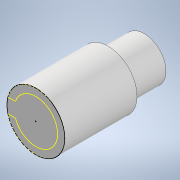
# Autodesk Inventor part: handle_base3
Saved by Autodesk Inventor 2021 (Build 250183000, 183)
## iProperties
Created: 2021-07-05
Part Number: handle_base3
Material: Generic
Document SubType Name: Modeling
Designer: teh18
Density: 1 g/cm^3
Appearance: Default
Author: teh18
Autodesk Inventor part; units mm, degrees
ref_plane "YZ Plane" through (0, 0, 0) normal (1, 0, 0) x (0, 1, 0)
ref_plane "XZ Plane" through (0, 0, 0) normal (0, 1, 0) x (-1, 0, 0)
ref_plane "XY Plane" through (0, 0, 0) normal (0, 0, 1) x (1, 0, 0)
sketch "Sketch1" plane through (0, 0, 0) normal (0, 0, 1) x (1, 0, 0)
  circle A0 centre (0, 0) radius 6.1 projected
  circle A1 centre (0, 0) radius 8 projected
  circle A2 centre (0, 0) radius 6.1 projected
  circle A3 centre (0, 0) radius 6
  circle A4 centre (-0.2369, 0.08) radius 5 projected
  circle A5 centre (-0.2369, 0.08) radius 5 projected
  point P0 (0, 0)
  dimension "d0" = 0.1
  constraints: 1 centre point
  measures "d0" radial gap between concentric circles of A0 A3
extrude "Extrusion1" add sketch "Sketch1" against normal blind 10 contours A3
sketch "Sketch2" plane through (0, 0, 0) normal (0, 0, 1) x (1, 0, 0)
  circle A0 centre (0, 0) radius 6.1 projected
  circle A1 centre (0, 0) radius 8 projected
  circle A2 centre (0, 0) radius 6 projected
  point P0 (0, 0)
extrude "Extrusion2" add sketch "Sketch2" along normal blind 20 contours A0 | A1
sketch "Sketch3" plane through (0, 0, 20) normal (0, 0, 1) x (1, 0, 0)
  line L0 (-1.3404, -2) -> (-8, -2)
  line L1 (-8, -2) -> (-8, 2)
  line L2 (-8, 2) -> (-1.3404, 2)
  line L3 (-1.3404, 2) -> (-1.3404, -2)
  line L4 (-1.3404, -2) -> (-8, 2) construction
  line L5 (-8, -2) -> (-1.3404, 2) construction
  point P0 (0, 0)
  point P1 (-4.6702, 0)
  dimension "d5" = 4
  constraints: 12 end point, 2 midpoint, 2 parallel, 1 horizontal, 1 perpendicular
  measures "d5" distance of L0.end L1.end
extrude "Extrusion3" cut sketch "Sketch3" against normal blind 7
sketch "Sketch4" plane through (0, 0, 20) normal (0, 0, 1) x (1, 0, 0)
  line L0 (-5.6569, -2) -> (-7.746, -2) projected
  arc A0 (-7.746, -2) -> (-7.746, 2) centre (0, 0) ccw projected
  line L1 (-7.746, 2) -> (-5.6569, 2) projected
  arc A1 (-5.6569, -2) -> (-5.6569, 2) centre (0, 0) ccw projected
  circle A2 centre (0, 0) radius 8
  point P0 (0, 0)
  point P1 (-7.746, 2)
  constraints: 1 centre point, 1 coincident, 1 concentric
extrude "Extrusion4" add sketch "Sketch4" against normal blind 3
sketch "Sketch6" plane through (0, 0, 20) normal (0, 0, 1) x (1, 0, 0)
  circle A0 centre (0, 0) radius 8 projected
  arc A1 (-4.1289, 4.2146) -> (-5.6926, 1.5507) centre (0, 0) ccw projected
  line L0 (-5.6926, 1.5507) -> (-7.0866, 0.985) projected
  line L1 (-7.0866, 0.985) -> (-5.8997, 0.0606) projected
  arc A2 (-5.8997, 0.0606) -> (-5.1217, -2.9288) centre (0, 0) ccw projected
  line L2 (-5.1217, -2.9288) -> (-5.7075, -4.3145) projected
  line L3 (-5.7075, -4.3145) -> (-4.2146, -4.1289) projected
  arc A3 (-4.2146, -4.1289) -> (-1.5507, -5.6926) centre (0, 0) ccw projected
  line L4 (-1.5507, -5.6926) -> (-0.985, -7.0866) projected
  line L5 (-0.985, -7.0866) -> (-0.0606, -5.8997) projected
  arc A4 (-0.0606, -5.8997) -> (2.9288, -5.1217) centre (0, 0) ccw projected
  line L6 (2.9288, -5.1217) -> (4.3145, -5.7075) projected
  line L7 (4.3145, -5.7075) -> (4.1289, -4.2146) projected
  arc A5 (4.1289, -4.2146) -> (5.6926, -1.5507) centre (0, 0) ccw projected
  line L8 (5.6926, -1.5507) -> (7.0866, -0.985) projected
  line L9 (7.0866, -0.985) -> (5.8997, -0.0606) projected
  arc A6 (5.8997, -0.0606) -> (5.1217, 2.9288) centre (0, 0) ccw projected
  line L10 (5.1217, 2.9288) -> (5.7075, 4.3145) projected
  line L11 (5.7075, 4.3145) -> (4.2146, 4.1289) projected
  arc A7 (4.2146, 4.1289) -> (1.5507, 5.6926) centre (0, 0) ccw projected
  line L12 (1.5507, 5.6926) -> (0.985, 7.0866) projected
  line L13 (0.985, 7.0866) -> (0.0606, 5.8997) projected
  arc A8 (0.0606, 5.8997) -> (-2.9288, 5.1217) centre (0, 0) ccw projected
  line L14 (-2.9288, 5.1217) -> (-4.3145, 5.7075) projected
  line L15 (-4.3145, 5.7075) -> (-4.1289, 4.2146) projected
  arc A9 (4.2351, -4.2514) -> (5.7765, -1.6254) centre (0, 0) ccw
  line L16 (4.2351, -4.2514) -> (4.4361, -5.8684)
  line L17 (4.4361, -5.8684) -> (2.9353, -5.234)
  arc A10 (-0.0115, -6.0008) -> (2.9353, -5.234) centre (0, 0) ccw
  line L18 (-0.0115, -6.0008) -> (-1.0128, -7.2864)
  line L19 (-1.0128, -7.2864) -> (-1.6254, -5.7765)
  arc A11 (-4.2514, -4.2351) -> (-1.6254, -5.7765) centre (0, 0) ccw
  line L20 (-4.2514, -4.2351) -> (-5.8684, -4.4361)
  line L21 (-5.8684, -4.4361) -> (-5.234, -2.9353)
  arc A12 (-6.0008, 0.0115) -> (-5.234, -2.9353) centre (0, 0) ccw
  line L22 (-6.0008, 0.0115) -> (-7.2864, 1.0128)
  line L23 (-7.2864, 1.0128) -> (-5.7765, 1.6254)
  arc A13 (-4.2351, 4.2514) -> (-5.7765, 1.6254) centre (0, 0) ccw
  line L24 (-4.2351, 4.2514) -> (-4.4361, 5.8684)
  line L25 (-4.4361, 5.8684) -> (-2.9353, 5.234)
  arc A14 (0.0115, 6.0008) -> (-2.9353, 5.234) centre (0, 0) ccw
  line L26 (0.0115, 6.0008) -> (1.0128, 7.2864)
  line L27 (1.0128, 7.2864) -> (1.6254, 5.7765)
  arc A15 (4.2514, 4.2351) -> (1.6254, 5.7765) centre (0, 0) ccw
  line L28 (4.2514, 4.2351) -> (5.8684, 4.4361)
  line L29 (5.8684, 4.4361) -> (5.234, 2.9353)
  arc A16 (6.0008, -0.0115) -> (5.234, 2.9353) centre (0, 0) ccw
  line L30 (6.0008, -0.0115) -> (7.2864, -1.0128)
  line L31 (7.2864, -1.0128) -> (5.7765, -1.6254)
  point P0 (0, 0)
  constraints: 32 end point, 16 point on circle, 8 centre point, 23 other
extrude "Extrusion5" cut sketch "Sketch6" against normal blind 2.1 contours L15 L14 A8 L13 L12 A7 L11 L10 A6 L9 L8 A5 L7 L6 A4 L5 L4 A3 L3 L2 A2 L1 L0 A1 | L16 L17 A10 L18 L19 A11 L20 L21 A12 L22 L23 A13 L24 L25 A14 L26 L27 A15 L28 L29 A16 L30 L31 A9
body "Solid1"
